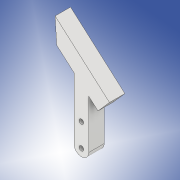
# Autodesk Inventor part: GA007
Saved by Autodesk Inventor 2017 (Build 210142000, 142)
## iProperties
Created: 2017-06-20
Part Number: GA007
Material: ABS Plastic
Document SubType Name: Modeling
Designer: zallen
Density: 1.06 g/cm^3
Appearance: CR White
Author: zallen
Autodesk Inventor part; units mm, degrees
ref_plane "YZ Plane" through (0, 0, 0) normal (1, 0, 0) x (0, 1, 0)
ref_plane "XZ Plane" through (0, 0, 0) normal (0, 1, 0) x (-1, 0, 0)
ref_plane "XY Plane" through (0, 0, 0) normal (0, 0, 1) x (1, 0, 0)
sketch "Sketch1" plane through (0, 0, 0) normal (0, 0, 1) x (1, 0, 0)
  line L0 (0, 0) -> (0, 40)
  circle A0 centre (4.75, 0) radius 4.75 construction
  line L1 (9.5, 0) -> (9.5, 31.654)
  arc A1 (0, 0) -> (9.5, 0) centre (4.75, 0) ccw
  line L2 (0, 40) -> (-11.269, 49.9)
  line L3 (9.5, 31.654) -> (15.5101, 26.374)
  line L4 (15.5101, 26.374) -> (22.9476, 34.84)
  line L5 (22.9476, 34.84) -> (-12.2974, 65.8035)
  line L6 (-12.2974, 65.8035) -> (-11.269, 49.9)
  circle A2 centre (4.75, 0) radius 1.5
  circle A3 centre (4.75, 15) radius 1.5
  line L7 (-11.269, 49.9) -> (16.1034, 25.8528) construction
  dimension "d0" = 40
  dimension "d1" = 9.5
  dimension "d3" = 15
  dimension "d4" = 8
  dimension "d6" = 3
  dimension "d7" = 3
  dimension "d8" = 15
  dimension "d13" = 131.3
  dimension "d21" = 90
  dimension "d23" = 11.269
  dimension "d24" = 135
  constraints: 16 end point, 4 centre point, 4 point on circle, 2 point on line, 2 tangent, 2 vertical, 1 coincident, 1 collinear, 1 horizontal alignment, 1 parallel, 1 vertical alignment
  measures "d0" distance of L0.start L0.end
  measures "d1" diameter of A0
  measures "d3" distance of L0.end L2.end
  measures "d4" distance of L1.end L3.end
  measures "d6" diameter of A2
  measures "d7" diameter of A3
  measures "d8" distance of A2.centre A3.centre
  measures "d13" angle of L2 L0
  measures "d21" angle of L4 L3
  measures "d23" distance of L3.end L4.end
  measures "d24" angle of L6 L7
extrude "Extrusion1" add sketch "Sketch1" along normal blind 10
body "Solid1"
